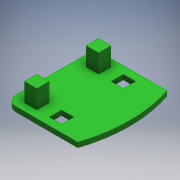
# Autodesk Inventor part: green_part
Saved by Autodesk Inventor 2016 (Build 200138000, 138)
## iProperties
Created: 2016-07-25
Part Number: green_part
Material: Plastique ABS
Document SubType Name: Modeling
Designer: tmonglon
Density: 1.06 g/cm^3
Appearance: Lisse - Vert forêt foncé
Author: tmonglon
Autodesk Inventor part; units mm, degrees
ref_plane "YZ Plane" through (0, 0, 0) normal (1, 0, 0) x (0, 1, 0)
ref_plane "XZ Plane" through (0, 0, 0) normal (0, 1, 0) x (-1, 0, 0)
ref_plane "XY Plane" through (0, 0, 0) normal (0, 0, 1) x (1, 0, 0)
sketch "Esquisse1" plane through (0, 0, 0) normal (0, 0, 1) x (1, 0, 0)
  line L0 (0, 0) -> (-29, 0)
  line L1 (-29, 0) -> (-29, 36)
  line L2 (-29, 36) -> (0, 36)
  line L3 (-24.5656, 33) -> (-19.5656, 33)
  line L4 (-19.5656, 33) -> (-19.5656, 28)
  line L5 (-19.5656, 28) -> (-24.5656, 28)
  line L6 (-24.5656, 28) -> (-24.5656, 33)
  line L7 (-14.5656, 33) -> (-9.5656, 33)
  line L8 (-9.5656, 33) -> (-9.5656, 28)
  line L9 (-9.5656, 28) -> (-14.5656, 28)
  line L10 (-14.5656, 28) -> (-14.5656, 33)
  line L11 (-24.5656, 8) -> (-19.5656, 8)
  line L12 (-19.5656, 8) -> (-19.5656, 3)
  line L13 (-19.5656, 3) -> (-24.5656, 3)
  line L14 (-24.5656, 3) -> (-24.5656, 8)
  line L15 (-14.5656, 8) -> (-9.5656, 8)
  line L16 (-9.5656, 8) -> (-9.5656, 3)
  line L17 (-9.5656, 3) -> (-14.5656, 3)
  line L18 (-14.5656, 3) -> (-14.5656, 8)
  arc A0 (0, 0) -> (0, 36) centre (-54.0833, 18) ccw
  dimension "d0" = 36
  dimension "d1" = 29
  dimension "d2" = 5
  dimension "d3" = 5
  dimension "d4" = 5
  dimension "d5" = 5
  dimension "d6" = 20
  dimension "d7" = 5
  dimension "d8" = 3
  dimension "d9" = 57
  constraints: 38 end point, 9 parallel, 8 point on line, 5 horizontal, 5 perpendicular, 2 point on circle, 1 centre point
  measures "d0" distance of L0.end L1.end
  measures "d1" distance of L1.end L2.end
  measures "d2" distance of L5.end L3.start
  measures "d3" distance of L3.start L3.end
  measures "d4" distance of L7.start L7.end
  measures "d5" distance between parallel lines of L10 L4
  measures "d6" distance between parallel lines of L15 L9
  measures "d7" distance of L15.end L16.end
  measures "d8" distance between parallel lines of L0 L17
  measures "d9" radius of A0
extrude "Extrusion1" add sketch "Esquisse1" along normal blind 2
extrude "Extrusion3" add sketch "Esquisse1" along normal blind 9.5 contours L3 L4 L5 L6 | L11 L12 L13 L14
fillet "Congé1" radius 4 2 edges at (-29, 0, 1) (-29, 36, 1)
